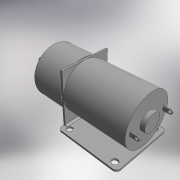
# Autodesk Inventor part: BallBallancing_DCmotor
Saved by Autodesk Inventor 2016 (Build 200138000, 138)
## iProperties
Created: 2016-04-08
Part Number: BallBallancing_DCmotor
Material: Generic
Document SubType Name: Modeling
Designer: Admin
Density: 1 g/cm^3
Appearance: Default
Author: Admin
Autodesk Inventor part; units mm, degrees
ref_plane "YZ Plane" through (0, 0, 0) normal (1, 0, 0) x (0, 1, 0)
ref_plane "XZ Plane" through (0, 0, 0) normal (0, 1, 0) x (-1, 0, 0)
ref_plane "XY Plane" through (0, 0, 0) normal (0, 0, 1) x (1, 0, 0)
sketch "Sketch1" plane through (0, 0, 0) normal (0, 0, 1) x (1, 0, 0)
  line L0 (-13.5, 15) -> (13.5, 15)
  line L1 (15.5, 13) -> (15.5, -13)
  line L2 (13.5, -15) -> (-13.5, -15)
  line L3 (-15.5, -13) -> (-15.5, 13)
  line L4 (-22.2799, 0) -> (22.2799, 0) projected
  line L5 (0, -21.5799) -> (0, 21.5799) projected
  circle A0 centre (-12, 12) radius 1.5
  arc A1 (-13.5, 15) -> (-15.5, 13) centre (-13.5, 13) ccw
  arc A2 (15.5, 13) -> (13.5, 15) centre (13.5, 13) ccw
  arc A3 (13.5, -15) -> (15.5, -13) centre (13.5, -13) ccw
  arc A4 (-15.5, -13) -> (-13.5, -15) centre (-13.5, -13) ccw
  circle A5 centre (12, 12) radius 1.5
  circle A6 centre (-12, -12) radius 1.5
  circle A7 centre (12, -12) radius 1.5
  point P0 (0, 0)
  point P1 (-15.5, 15)
  point P2 (15.5, -15)
  point P3 (15.5, 15)
  point P4 (13.5, 13)
  dimension "d0" = 31
  dimension "d1" = 30
  dimension "d2" = 15
  dimension "d3" = 15.5
  dimension "d4" = 3
  dimension "d5" = 12
  dimension "d6" = 12
  dimension "d7" = 2
  constraints: 8 centre point, 8 end point, 8 point on circle, 8 tangent, 6 point on line, 4 symmetric about line, 3 equal radius, 2 parallel, 1 horizontal, 1 perpendicular, 3 other
  measures "d0" distance of point (-15.5, 15) point (15.5, 15)
  measures "d1" distance of point (15.5, 15) point (15.5, -15)
  measures "d2" distance between parallel lines of L4 L0
  measures "d3" distance between parallel lines of L5 L1
  measures "d4" diameter of A0
  measures "d5" distance from line of L5 A0.centre
  measures "d6" distance from line of L4 A0.centre
  measures "d7" radius of A1
extrude "Extrusion1" add sketch "Sketch1" along normal blind 0.9
sketch "Sketch2" plane through (0, 0, 0.9) normal (0, 0, 1) x (1, 0, 0)
  circle A0 centre (12, -12) radius 1.5 projected
  circle A1 centre (-12, -12) radius 1.5 projected
  circle A2 centre (12, 12) radius 1.5 projected
  circle A3 centre (-12, 12) radius 1.5 projected
  line L0 (13.5, 15) -> (-13.5, 15) projected
  arc A4 (-13.5, 15) -> (-15.5, 13) centre (-13.5, 13) ccw projected
  line L1 (-15.5, 13) -> (-15.5, -13) projected
  arc A5 (-15.5, -13) -> (-13.5, -15) centre (-13.5, -13) ccw projected
  line L2 (-13.5, -15) -> (13.5, -15) projected
  arc A6 (13.5, -15) -> (15.5, -13) centre (13.5, -13) ccw projected
  line L3 (15.5, -13) -> (15.5, 13) projected
  arc A7 (15.5, 13) -> (13.5, 15) centre (13.5, 13) ccw projected
  line L4 (-15.5, 12) -> (-14.6, 12)
  line L5 (-14.6, 12) -> (-14.6, -12)
  line L6 (-14.6, -12) -> (-15.5, -12)
  line L7 (-15.5, -12) -> (-15.5, 12)
  line L8 (-22.2799, 0) -> (22.2799, 0) projected
  line L9 (0, -21.5799) -> (0, 21.5799) projected
  point P0 (0, 0)
  dimension "d10" = 0.9
  dimension "d11" = 24
  dimension "d12" = 12
  constraints: 8 end point, 2 parallel, 1 horizontal, 1 perpendicular, 1 point on line
  measures "d10" distance between parallel lines of L1 L5
  measures "d11" distance between parallel lines of L4 L6
  measures "d12" distance between parallel lines of L8 L4
extrude "Extrusion2" add sketch "Sketch2" along normal blind 26.1 contours L8 L1 L4 L5 | L5 L6 L1 L8
fillet "Fillet1" radius 1 1 edges at (-14.6, 0, 0.9)
sketch "Sketch3" plane through (-14.6, -12, 27) normal (1, 0, 0) x (0, 0, -1)
  line L0 (27, -1) -> (27, 25) projected
  line L1 (27, -1) -> (26.1, -1) projected
  line L2 (26.1, 0) -> (26.1, -1) projected
  line L3 (26.1, 0) -> (0, 0) projected
  line L4 (0, 24) -> (0, 0) projected
  line L5 (26.1, 24) -> (0, 24) projected
  line L6 (26.1, 25) -> (26.1, 24) projected
  line L7 (27, 25) -> (26.1, 25) projected
  line L8 (35.3744, 12) -> (2.9643, 12) construction
  circle A0 centre (12, 12) radius 12
  point P0 (27, 12)
  dimension "d16" = 15
  dimension "d17" = 24
  constraints: 2 end point, 1 centre point, 1 horizontal, 1 point on line
  measures "d16" distance from line of L0 A0.centre
  measures "d17" diameter of A0
extrude "Extrusion3" add sketch "Sketch3" along normal blind 30.1 contours A0
sketch "Sketch4" plane through (-15.5, -13, 0) normal (-1, 0, 0) x (0, 0, 1)
  circle A0 centre (15, 13) radius 12 projected
  arc A1 (15, 25) -> (15, 1) centre (15, 13) ccw projected
  arc A2 (27, 13) -> (15, 25) centre (15, 13) ccw projected
  arc A3 (15, 1) -> (27, 13) centre (15, 13) ccw projected
  circle A4 centre (15, 13) radius 12.5
  point P0 (0, 13)
  dimension "d20" = 25
  constraints: 1 centre point, 1 coincident
  measures "d20" diameter of A4
extrude "Extrusion4" add sketch "Sketch4" along normal blind 16.5 contours A0 | A4
sketch "Sketch5" plane through (15.5, 0, 15) normal (1, 0, 0) x (0, 0, -1)
  circle A0 centre (0, 0) radius 12 projected
  arc A1 (0, -12) -> (0, 12) centre (0, 0) ccw projected
  arc A2 (0, 12) -> (-12, 0) centre (0, 0) ccw projected
  arc A3 (-12, 0) -> (0, -12) centre (0, 0) ccw projected
  circle A4 centre (0, 0) radius 4.25
  point P0 (15, 0)
  dimension "d23" = 8.5
  constraints: 1 centre point, 1 coincident
  measures "d23" diameter of A4
extrude "Extrusion5" add sketch "Sketch5" along normal blind 2 contours A4
sketch "Sketch6" plane through (15.5, 0, 15) normal (1, 0, 0) x (0, 0, -1)
  circle A0 centre (0, 0) radius 12 projected
  arc A1 (0, -12) -> (0, 12) centre (0, 0) ccw projected
  arc A2 (0, 12) -> (-12, 0) centre (0, 0) ccw projected
  arc A3 (-12, 0) -> (0, -12) centre (0, 0) ccw projected
  line L0 (0, 12.481) -> (0, -10.3275) construction
  line L1 (-1, -9.75) -> (1, -9.75)
  line L2 (1, -9.75) -> (1, -9.25)
  line L3 (1, -9.25) -> (-1, -9.25)
  line L4 (-1, -9.25) -> (-1, -9.75)
  line L5 (0, 0) -> (-4.6495, 0) construction
  line L6 (-1, 9.75) -> (1, 9.75)
  line L7 (1, 9.75) -> (1, 9.25)
  line L8 (1, 9.25) -> (-1, 9.25)
  line L9 (-1, 9.25) -> (-1, 9.75)
  point P0 (15, 0)
  point P1 (0, 10.3275)
  dimension "d26" = 2
  dimension "d27" = 1
  dimension "d28" = 0.5
  dimension "d29" = 9.25
  constraints: 20 end point, 5 symmetric about line, 2 horizontal, 2 parallel, 1 perpendicular, 1 point on line, 1 vertical
  measures "d26" distance between parallel lines of L4 L2
  measures "d27" distance between parallel lines of L0 L2
  measures "d28" distance between parallel lines of L3 L1
  measures "d29" distance from line of A0.centre L3
extrude "Extrusion6" add sketch "Sketch6" along normal blind 4 contours L4 L3 L2 L1 | L6 L7 L8 L9
sketch "Sketch7" plane through (15.5, -9.75, 14) normal (0, -1, 0) x (1, 0, 0)
  line L0 (0, 0) -> (0, 2) projected
  line L1 (0, 0) -> (4, 0) projected
  line L2 (4, 2) -> (4, 0) projected
  line L3 (0, 2) -> (4, 2) projected
  line L4 (4, 1) -> (0, 1) construction
  line L5 (0, 0) -> (0, 2) projected
  circle A0 centre (2.95, 1) radius 0.75
  point P0 (-15.5, -14)
  dimension "d32" = 1.5
  dimension "d33" = 1.05
  constraints: 2 end point, 2 midpoint, 1 centre point, 1 point on line
  measures "d32" diameter of A0
  measures "d33" distance from line of L2 A0.centre
extrude "Extrusion7" cut sketch "Sketch7" against normal through all contours A0
fillet "Fillet2" radius 1 2 edges at (19.5, -9.5, 16) (19.5, -9.5, 14)
fillet "Fillet3" radius 1 2 edges at (19.5, 9.5, 16) (19.5, 9.5, 14)
sketch "Sketch8" plane through (-32, 0, 15) normal (-1, 0, 0) x (0, 0, 1)
  circle A0 centre (0, 0) radius 12.5 projected
  circle A1 centre (0, 0) radius 2.485
  point P0 (-15, 0)
  dimension "d38" = 4.97
  constraints: 1 centre point, 1 coincident
  measures "d38" diameter of A1
extrude "Extrusion8" add sketch "Sketch8" along normal blind 6 contours A1
sketch "Sketch9" plane through (-38, 0, 15) normal (-1, 0, 0) x (0, 0, 1)
  circle A0 centre (0, 0) radius 2.485 projected
  circle A1 centre (0, 0) radius 0.99
  point P0 (-15, 0)
  dimension "d41" = 1.98
  constraints: 1 centre point, 1 coincident
  measures "d41" diameter of A1
extrude "Extrusion9" add sketch "Sketch9" along normal blind 6.5 contours A1
sketch "Sketch10" plane through (0, 0, 0) normal (0, 1, 0) x (-1, 0, 0)
  line L0 (44.5, 14.01) -> (44.5, 15.99) projected
  line L1 (38, 15.99) -> (38, 14.01) projected
  line L2 (42, 15.99) -> (39, 15.99)
  line L3 (39, 15.99) -> (39, 15.49)
  line L4 (39, 15.49) -> (42, 15.49)
  line L5 (42, 15.49) -> (42, 15.99)
  line L6 (38, 15.99) -> (44.5, 15.99) construction
  line L7 (38, 15.99) -> (44.5, 15.99) projected
  point P0 (0, 0)
  dimension "d44" = 3
  dimension "d45" = 0.5
  dimension "d46" = 1
  constraints: 10 end point, 3 equal length, 1 collinear, 1 horizontal, 1 perpendicular
  measures "d44" distance of L3.end L4.end
  measures "d45" distance between parallel lines of L2 L4
  measures "d46" distance between parallel lines of L1 L3
extrude "Extrusion10" cut sketch "Sketch10" along normal mid plane 6.5
equation "\"d2\" = 0.5 * d1"
equation "\"d3\" = 0.5 * d0"
equation "\"d12\" = 0.5 * d11"
equation "\"d27\" = 0.5 * d26"
body "Solid1"
